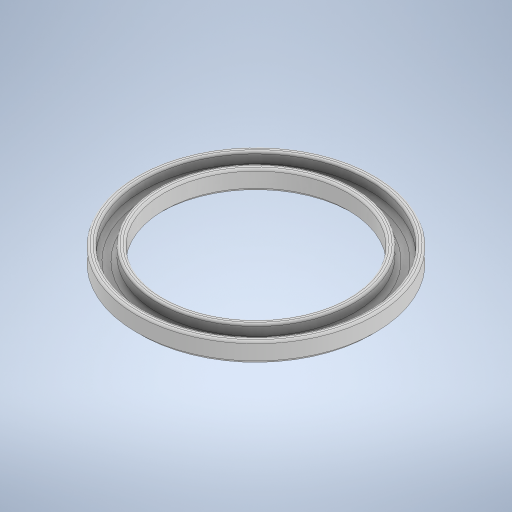
# Autodesk Inventor part: LN2-Dish-SuperconductingSolenoid
Saved by Autodesk Inventor 2023 (Build 270158000, 158)
## iProperties
Created: 2024-05-05
Part Number: LN2-Dish-SuperconductingSolenoid
Material: Generic
Document SubType Name: Modeling
Designer: incep
Density: 1 g/cm^3
Appearance: Default
Author: incep
## iProperties of the stored document LN2-Dish-SuperconductingSolenoid_3DPrint.ipt
Created: 2024-05-05
Part Number: LN2-Dish-SuperconductingSolenoid_3DPrint
Material: Generic
Document SubType Name: Modeling
Designer: incep
Density: 1 g/cm^3
Appearance: Default
Author: incep
Autodesk Inventor part; units mm, degrees
ref_plane "YZ Plane" through (0, 0, 0) normal (1, 0, 0) x (0, 1, 0)
ref_plane "XZ Plane" through (0, 0, 0) normal (0, 1, 0) x (-1, 0, 0)
ref_plane "XY Plane" through (0, 0, 0) normal (0, 0, 1) x (1, 0, 0)
sketch "Sketch1" plane through (0, 0, 0) normal (0, 1, 0) x (-1, 0, 0)
  circle A0 centre (0, 0) radius 50 construction
  circle A1 centre (0, 0) radius 46.5
  circle A2 centre (0, 0) radius 53.5
  circle A3 centre (0, 0) radius 43.5
  circle A4 centre (0, 0) radius 56.5
  dimension "d0" = 3.5
  dimension "d1" = 100
  dimension "d2" = 3.5
  dimension "d3" = 3
  dimension "d4" = 3
  constraints: 5 centre point, 1 coincident
  measures "d0" radial gap between concentric circles of A0 A1
  measures "d1" diameter of A0
  measures "d2" radial gap between concentric circles of A0 A2
  measures "d3" radial gap between concentric circles of A1 A3
  measures "d4" radial gap between concentric circles of A2 A4
extrude "Extrusion1" add sketch "Sketch1" against normal blind 3 contours A1 | A2 | A3 | A4
extrude "Extrusion2" cut sketch "Sketch1" against normal blind 3 contours A3
extrude "Extrusion3" add sketch "Sketch1" along normal blind 7
fillet "Fillet1" radius 2 2 edges at (53.5, 0, 0) (46.5, 0, 0)
chamfer "Chamfer1" distance 2 angle 45 2 edges at (43.5, -3, 0) (56.5, -3, 0)
fillet "Fillet2" radius 1 4 edges at (43.5, 7, 0) (46.5, 7, 0) (56.5, 7, 0) (53.5, 7, 0)
body "Solid1"
